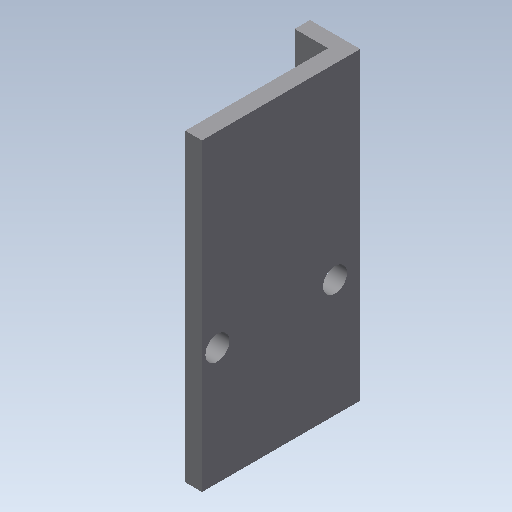
# Autodesk Inventor part: allignment plate
Saved by Autodesk Inventor 2020 (Build 240168000, 168)
## iProperties
Created: 2016-07-14
Part Number: allignment plate
Material: Generic
Document SubType Name: Modeling
Designer: labuser
Density: 1 g/cm^3
Appearance: Default
Author: labuser
Autodesk Inventor part; units mm, degrees
ref_plane "YZ Plane" through (0, 0, 0) normal (1, 0, 0) x (0, 1, 0)
ref_plane "XZ Plane" through (0, 0, 0) normal (0, 1, 0) x (-1, 0, 0)
ref_plane "XY Plane" through (0, 0, 0) normal (0, 0, 1) x (1, 0, 0)
sketch "Sketch1" plane through (0, 0, 0) normal (1, 0, 0) x (0, 1, 0)
  line L0 (0, 0) -> (57.7088, 0)
  line L1 (57.7088, 0) -> (57.7088, 29.9974)
  line L2 (57.7088, 29.9974) -> (0, 29.9974)
  line L3 (0, 29.9974) -> (0, 0)
  circle A0 centre (22.225, 27.0764) radius 2.286
  circle A1 centre (22.225, 4.7752) radius 2.286
  dimension "d0" = 57.7088
  dimension "d1" = 29.9974
  dimension "d2" = 4.572
  dimension "d3" = 2.921
  dimension "d4" = 22.225
  dimension "d5" = 4.572
  dimension "d6" = 22.225
  dimension "d7" = 25.2222
  constraints: 8 end point, 2 centre point, 2 parallel, 1 horizontal, 1 perpendicular
  measures "d0" distance of L2.end L1.end
  measures "d1" distance of L1.end L0.end
  measures "d2" diameter of A0
  measures "d3" distance from line of A0.centre L2
  measures "d4" distance from line of L3 A0.centre
  measures "d5" diameter of A1
  measures "d6" distance from line of A1.centre L3
  measures "d7" distance from line of L2 A1.centre
extrude "Extrusion1" add sketch "Sketch1" along normal blind 3.175
sketch "Sketch2" plane through (0, 0, 0) normal (-1, 0, 0) x (0, 0, 1)
  line L0 (0, 57.7088) -> (2.921, 57.7088)
  line L1 (2.921, 57.7088) -> (2.921, 29.7688)
  line L2 (2.921, 29.7688) -> (0, 29.7688)
  line L3 (0, 29.7688) -> (0, 57.7088)
  dimension "d10" = 2.921
  dimension "d11" = 27.94
  constraints: 8 end point, 2 parallel, 1 horizontal, 1 perpendicular
  measures "d10" distance of L1.end L2.end
  measures "d11" distance of L0.end L1.end
extrude "Extrusion2" add sketch "Sketch2" along normal blind 6.35
sketch "Sketch3" plane through (0, 29.7688, 2.921) normal (0, 0, 1) x (1, 0, 0)
  line L0 (0, 27.94) -> (0, 0) projected
  line L1 (-6.35, 27.94) -> (0, 27.94)
  line L2 (0, 27.94) -> (0, 16.51)
  line L3 (0, 16.51) -> (-6.35, 16.51)
  line L4 (-6.35, 16.51) -> (-6.35, 27.94)
  point P0 (0, -29.7688)
  dimension "d14" = 11.43
  constraints: 8 end point, 2 parallel, 1 horizontal, 1 perpendicular, 1 point on line
  measures "d14" distance of L1.end L2.end
extrude "Extrusion3" [suppressed]
body "Solid1"
